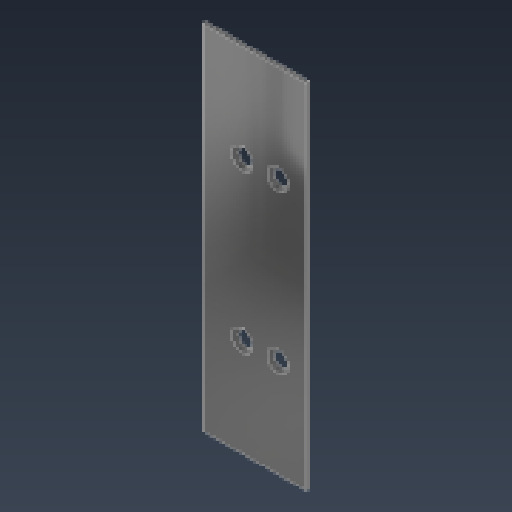
# Autodesk Inventor part: MetalBack
Saved by Autodesk Inventor 2027.1 (Build 311270010, 270A)
## iProperties
Created: 2026-05-03
Part Number: MetalBack
Material: Stainless Steel
Document SubType Name: Modeling
Designer: szymo
Density: 8 g/cm^3
Appearance: Aluminum - Flat(2)
Mass: 23.2938 g
Surface Area: 61.1995 cm^2
Volume: 2.91173 cm^3
Author: szymo
Autodesk Inventor part; units mm, degrees
ref_plane "YZ Plane" through (0, 0, 0) normal (1, 0, 0) x (0, 1, 0)
ref_plane "XZ Plane" through (0, 0, 0) normal (0, 1, 0) x (-1, 0, 0)
ref_plane "XY Plane" through (0, 0, 0) normal (0, 0, 1) x (1, 0, 0)
sketch "Sketch1" plane through (0, 0, 0) normal (0, 0, 1) x (1, 0, 0)
  line L0 (0, -50) -> (-29.4, -50)
  line L1 (-29.4, -50) -> (-29.4, 50)
  line L2 (-29.4, 50) -> (0, 50)
  line L3 (0, 50) -> (0, -50)
  line L4 (0, -13.95) -> (-29.4, -13.95) projected
  point P0 (0, 0)
  dimension "d0" = 50
  dimension "d1" = 50
  dimension "d2" = 0
  constraints: 8 end point, 2 parallel, 1 horizontal, 1 midpoint, 1 perpendicular
  measures "d0" distance from line of L0 point (0, 0)
  measures "d1" distance from line of point (0, 0) L2
  measures "d2" distance from line of L1 L4.end
extrude "Extrusion1" add sketch "Sketch1" along normal blind 1
sketch "Sketch2" plane through (0, 0, 1) normal (0, 0, 1) x (1, 0, 0)
  circle A0 centre (-8.025, -22.2) radius 1.425 projected
  circle A1 centre (-18.075, -22.2) radius 1.425 projected
  line L0 (-27.4, -19.2) -> (0, -19.2) projected
  line L1 (-27.4, -19.2) -> (-27.4, -28.5) projected
  line L2 (-27.4, -28.5) -> (0, -28.5) projected
  line L3 (0, -19.2) -> (0, -28.5) projected
  circle A2 centre (-8.025, 22.45) radius 1.2295 projected
  circle A3 centre (-18.075, 22.45) radius 1.2295 projected
  line L4 (-27.4, 19.2) -> (0, 19.2) projected
  line L5 (0, 19.2) -> (0, 28.5) projected
  line L6 (0, 28.5) -> (-27.4, 28.5) projected
  line L7 (-27.4, 19.2) -> (-27.4, 28.5) projected
  point P0 (0, 0)
hole "Hole1" at (-8.025, -22.2, 1) at (-18.075, -22.2, 1) at (-18.075, 22.45, 1) at (-8.025, 22.45, 1) direction (0, 0, -1) diameter 3 depth 10 countersink diameter 6 countersink angle 90
body "Solid1"
